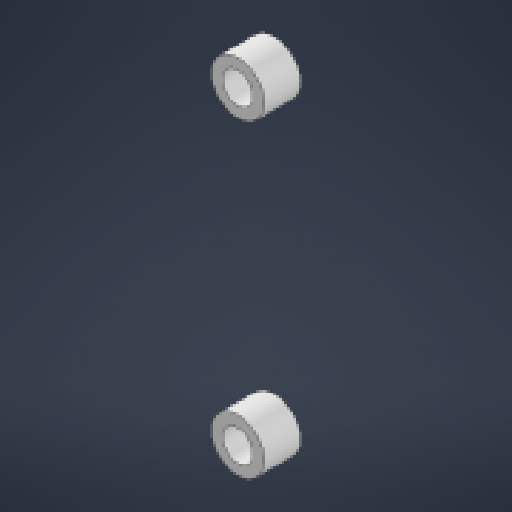
# Autodesk Inventor part: i2c_mplx_spacer
Saved by Autodesk Inventor 2024 (Build 280153000, 153)
## iProperties
Created: 2026-03-30
Part Number: i2c_mplx_spacer
Material: Generic
Document SubType Name: Modeling
Designer: schar
Density: 1 g/cm^3
Appearance: Default
Author: schar
Autodesk Inventor part; units mm, degrees
ref_plane "YZ Plane" through (0, 0, 0) normal (1, 0, 0) x (0, 1, 0)
ref_plane "XZ Plane" through (0, 0, 0) normal (0, 1, 0) x (-1, 0, 0)
ref_plane "XY Plane" through (0, 0, 0) normal (0, 0, 1) x (1, 0, 0)
sketch "Sketch1" plane through (0, 0, 0) normal (0, 0, 1) x (1, 0, 0)
  circle A0 centre (50.533, 12.7) radius 1.27 projected
  circle A1 centre (50.533, -12.7) radius 1.27 projected
  circle A2 centre (50.533, 12.7) radius 2.159
  circle A3 centre (50.533, -12.7) radius 2.159
  point P0 (0, 0)
  dimension "d0" = 4.318
  dimension "d1" = 4.318
  constraints: 2 centre point, 2 coincident
  measures "d0" diameter of A2
  measures "d1" diameter of A3
extrude "Extrusion1" add sketch "Sketch1" along normal blind 2.9997
body "Solid1"
